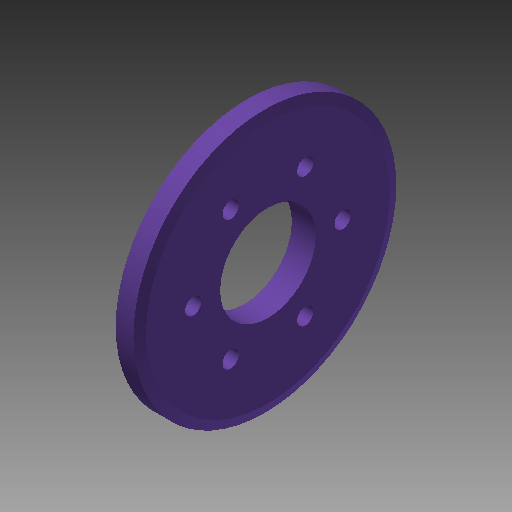
# Autodesk Inventor part: CHA_005_DrivePulleyCenterFlange
Saved by Autodesk Inventor 2018 (Build 220112000, 112)
## iProperties
Created: 2016-01-27
Part Number: CHA_005_DrivePulleyCenterFlange
Material: ABS Plastic
Document SubType Name: Modeling
Designer: Katelyn Angeliu
Density: 1.06 g/cm^3
Appearance: Violet
Mass: 10.9044 g
Surface Area: 54.9586 cm^2
Volume: 10.2872 cm^3
Author: Katelyn Angeliu
Autodesk Inventor part; units mm, degrees
ref_plane "YZ Plane" through (0, 0, 0) normal (1, 0, 0) x (0, 1, 0)
ref_plane "XZ Plane" through (0, 0, 0) normal (0, 1, 0) x (-1, 0, 0)
ref_plane "XY Plane" through (0, 0, 0) normal (0, 0, 1) x (1, 0, 0)
sketch "Sketch1" plane through (0, 0, 0) normal (1, 0, 0) x (0, 1, 0)
  circle A0 centre (0, 0) radius 27.94
  dimension "d0" = 55.88
  constraints: 1 centre point, 1 coincident
  measures "d0" diameter of A0
extrude "Extrusion1" add sketch "Sketch1" along normal blind 5.08
sketch "Sketch3" plane through (5.08, 0, 0) normal (1, 0, 0) x (0, 0, -1)
  point P0 (0, 0)
  point P1 (15.875, 0)
  dimension "d6" = 15.875
  measures "d6" distance of point (15.875, 0) point (0, 0)
hole "Hole1" at (5.08, 0, -15.875) direction (-1, 0, 0) diameter 3.5052 end through all
pattern_circular "Circular Pattern1" count 6 over 360 about axis through (-10, 0, 0) along (1, 0, 0) of "Hole1"
chamfer "Chamfer1" distance 2.032 angle 18 1 edges at (0, -27.94, 0) measured on face at (0, 4.0768, 2.3537)
sketch "Sketch4" plane through (5.08, 0, 0) normal (1, 0, 0) x (0, 0, -1)
  circle A0 centre (0, 0) radius 10.16
  dimension "d20" = 20.32
  constraints: 1 centre point, 1 coincident
  measures "d20" diameter of A0
extrude "Extrusion3" cut sketch "Sketch4" against normal through all
chamfer "Chamfer2" distance 2.032 angle 18 1 edges at (5.08, -27.94, 0) measured on face at (5.08, -19.1807, 0)
body "Solid1"
